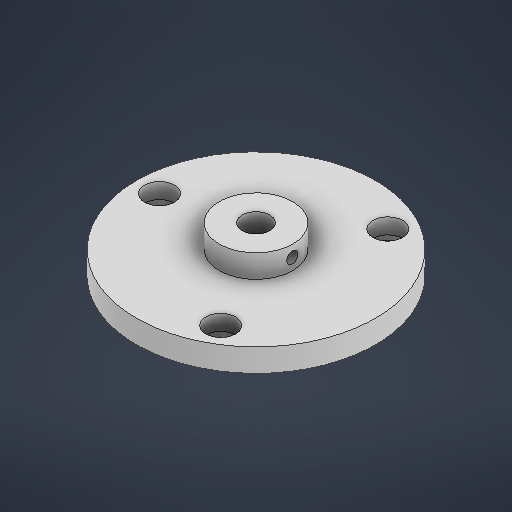
# Autodesk Inventor part: rotation stopper
Saved by Autodesk Inventor 2025.2 (Build 292293000, 293)
## iProperties
Created: 2025-06-02
Part Number: rotation stopper
Material: Generic
Document SubType Name: Modeling
Designer: klawy
Density: 1 g/cm^3
Appearance: Default
Author: klawy
Autodesk Inventor part; units mm, degrees
ref_plane "XZ Plane" through (0, 0, 0) normal (0, 1, 0) x (-1, 0, 0)
sketch "Sketch1" plane through (0, 0, 0) normal (0, 1, 0) x (-1, 0, 0)
  circle A0 centre (0, 0) radius 10
  circle A1 centre (0, 0) radius 26
  dimension "d0" = 20
  dimension "d8" = 52
  constraints: 2 centre point, 2 coincident
  measures "d0" diameter of A0
  measures "d8" diameter of A1
extrude "Extrusion1" add sketch "Sketch1" along normal blind 5
sketch "Sketch2" plane through (0, 0, 0) normal (0, -1, 0) x (1, 0, 0)
  circle A0 centre (0, 0) radius 14
  circle A1 centre (0, 0) radius 10 projected
  dimension "d56" = 28
  constraints: 1 centre point, 1 coincident
  measures "d56" diameter of A0
extrude "Extrusion2" add sketch "Sketch2" along normal blind 2.5
sketch "Sketch3" plane through (0, 5, 0) normal (0, 1, 0) x (1, 0, 0)
  circle A0 centre (0, 0) radius 21 construction
  line L0 (36.4, 0) -> (-36.4, 0) projected
  circle A1 centre (0, 0) radius 21 construction
  circle A2 centre (0, 0) radius 21 construction
  point P0 (-21, 0)
  point P1 (10.5, -18.1865)
  point P2 (10.5, 18.1865)
  dimension "d7" = 42
  dimension "d11" = 360
  constraints: 1 coincident, 1 horizontal alignment, 1 point on line, 18 other
hole "Hole1" at (-21, 5, 0) at (10.5, 5, 18.1865) at (10.5, 5, -18.1865) direction (0, -1, 0) diameter 3.4 end through all counterbore diameter 6.5 counterbore depth 3.4 clearance for "Socket Head Cap Screw ISO 4762" size "M3" standard "ISO"
ref_plane "Work Plane2" through (0, 1, 0) normal (0, -1, 0) x (1, 0, 0)
sketch "Sketch8" plane through (0, 1, 0) normal (0, -1, 0) x (1, 0, 0)
  circle A0 centre (0, 0) radius 10 projected
  circle A1 centre (0, 0) radius 10 projected
  circle A2 centre (0, 0) radius 3
  dimension "d39" = 6
  constraints: 1 centre point, 1 coincident
  measures "d39" diameter of A2
extrude "Extrusion5" add sketch "Sketch8" against normal blind 9
ref_plane "Work Plane3" through (8, 0, 0) normal (1, 0, 0) x (0, 1, 0)
sketch "Sketch9" plane through (0, 10, 0) normal (0, 1, 0) x (1, 0, 0)
  circle A0 centre (0, 0) radius 8
  circle A1 centre (0, 0) radius 3 projected
  circle A2 centre (0, 0) radius 10 projected
  circle A3 centre (0, 0) radius 3 projected
  dimension "d43" = 5
  constraints: 1 centre point, 1 coincident
  measures "d43" radial gap between concentric circles of A1 A0
extrude "Extrusion6" cut sketch "Sketch9" against normal blind 5 contours A2
sketch "Sketch10" plane through (8, 0, 0) normal (1, 0, 0) x (0, 1, 0)
  line L0 (5, -8) -> (5, 8) projected
  line L1 (10, -8) -> (10, 8) projected
  line L2 (10, 0) -> (5, 0) construction
  point P0 (0, 0)
  point P1 (7.5, 0)
  constraints: 3 midpoint, 2 end point
hole "Hole3" at (8, 7.5, 0) direction (-1, 0, 0) diameter 2.459 depth 8.8 tip angle 118 thread size "M3x0.5" class "6H" standard "ISO Metric profile"
chamfer "Chamfer1" distance 0.5 angle 45 1 edges at (-14, -2.5, 0)
body "Solid1"
